Autodesk Fusion 360 part; units mm, degrees
(part 12 of 18)
sketch "Sketch4" plane through (0, 0, 3) normal (0, 0, 1) x (-1, 0, 0)
  arc A0 (-3.0787, 1.9914) -> (-3.5852, 0.7688) centre (0, 0) ccw
  line L0 (-3.5852, 0.7688) -> (-4.9003, 1.0509)
  line L1 (-4.9003, 1.0509) -> (-4.9011, 1.051)
  spline S0 degree 5 poles (-4.9011, 1.051) (-4.9011, 1.0511) (-4.9013, 1.0511) (-4.9016, 1.0512) (-4.9021, 1.0512) (-4.9028, 1.0514) (-4.9036, 1.0515) (-4.9045, 1.0517) (-4.9055, 1.0518) (-4.9066, 1.052) (-4.9078, 1.0522) (-4.9092, 1.0524) (-4.9106, 1.0526) (-4.9121, 1.0529) (-4.9137, 1.0531) (-4.9154, 1.0533) (-4.9172, 1.0536) (-4.9191, 1.0538) (-4.9211, 1.054) (-4.9232, 1.0543) (-4.9254, 1.0545) (-4.9277, 1.0548) (-4.9301, 1.055) (-4.9325, 1.0553) (-4.9351, 1.0555) (-4.9377, 1.0558) (-4.9404, 1.056) (-4.9432, 1.0562) (-4.9461, 1.0564) (-4.9491, 1.0567) (-4.9521, 1.0569) (-4.9553, 1.0571) (-4.9585, 1.0573) (-4.9618, 1.0575) (-4.9652, 1.0576) (-4.9687, 1.0578) (-4.9722, 1.058) (-4.9758, 1.0581) (-4.9795, 1.0582) (-4.9833, 1.0583) (-4.9872, 1.0584) (-4.9911, 1.0585) (-4.9951, 1.0586) (-4.9992, 1.0587) (-5.0033, 1.0587) (-5.0075, 1.0587) (-5.0118, 1.0587) (-5.0162, 1.0587) (-5.0206, 1.0587) (-5.0251, 1.0587) (-5.0297, 1.0586) (-5.0344, 1.0585) (-5.0391, 1.0584) (-5.0439, 1.0583) (-5.0487, 1.0581) (-5.0536, 1.058) (-5.0586, 1.0578) (-5.0637, 1.0576) (-5.0688, 1.0573) (-5.074, 1.0571) (-5.0792, 1.0568) (-5.0845, 1.0565) (-5.0899, 1.0561) (-5.0953, 1.0558) (-5.1008, 1.0554) (-5.1063, 1.055) (-5.112, 1.0545) (-5.1176, 1.0541) (-5.1234, 1.0536) (-5.1291, 1.0531) (-5.135, 1.0525) (-5.1409, 1.0519) (-5.1469, 1.0513) (-5.1529, 1.0507) (-5.159, 1.05) (-5.1651, 1.0493) (-5.1713, 1.0486) (-5.1775, 1.0479) (-5.1838, 1.0471) (-5.1902, 1.0463) (-5.1966, 1.0454) (-5.203, 1.0446) (-5.2095, 1.0436) (-5.2161, 1.0427) (-5.2227, 1.0417) (-5.2294, 1.0407) (-5.2361, 1.0397) (-5.2428, 1.0386) (-5.2496, 1.0375) (-5.2565, 1.0364) (-5.2634, 1.0352) (-5.2704, 1.034) (-5.2774, 1.0327) (-5.2844, 1.0314) (-5.2915, 1.0301) (-5.2987, 1.0288) (-5.3059, 1.0274) (-5.3131, 1.026) (-5.3204, 1.0245) (-5.3277, 1.023) (-5.3351, 1.0215) (-5.3425, 1.0199) (-5.3499, 1.0183) (-5.3574, 1.0167) (-5.365, 1.015) (-5.3726, 1.0133) (-5.3802, 1.0115) (-5.3879, 1.0097) (-5.3956, 1.0079) (-5.4033, 1.006) (-5.4111, 1.0041) (-5.4189, 1.0021) (-5.4268, 1.0001) (-5.4347, 0.9981) (-5.4427, 0.996) (-5.4506, 0.9939) (-5.4587, 0.9918) (-5.4667, 0.9896) (-5.4748, 0.9874) (-5.483, 0.9851) (-5.4911, 0.9828) (-5.4993, 0.9804) (-5.5076, 0.978) (-5.5159, 0.9756) (-5.5242, 0.9731) (-5.5325, 0.9706) (-5.5409, 0.968) (-5.5493, 0.9654) (-5.5577, 0.9628) (-5.5662, 0.9601) (-5.5747, 0.9574) (-5.5833, 0.9546) (-5.5919, 0.9518) (-5.6005, 0.9489) (-5.6091, 0.946) (-5.6178, 0.9431) (-5.6265, 0.9401) (-5.6352, 0.9371) (-5.644, 0.934) (-5.6528, 0.9309) (-5.6616, 0.9277) (-5.6704, 0.9245) (-5.6793, 0.9213) (-5.6882, 0.918) (-5.6971, 0.9146) (-5.7061, 0.9113) (-5.7151, 0.9078) (-5.7241, 0.9044) (-5.7331, 0.9008) (-5.7422, 0.8973) (-5.7513, 0.8937) (-5.7604, 0.89) (-5.7695, 0.8863) (-5.7787, 0.8826) (-5.7879, 0.8788) (-5.7971, 0.875) (-5.8063, 0.8711) (-5.8156, 0.8672) (-5.8249, 0.8632) (-5.8342, 0.8592) (-5.8435, 0.8551) (-5.8529, 0.851) (-5.8622, 0.8469) (-5.8716, 0.8427) (-5.881, 0.8384) (-5.8905, 0.8341) (-5.8999, 0.8298) (-5.9094, 0.8254) (-5.9189, 0.821) (-5.9284, 0.8165) (-5.938, 0.812) (-5.9475, 0.8074) (-5.9571, 0.8028) (-5.9667, 0.7981) (-5.9763, 0.7934) (-5.9859, 0.7887) (-5.9956, 0.7839) (-6.0052, 0.779) (-6.0149, 0.7741) (-6.0246, 0.7692) (-6.0343, 0.7642) (-6.044, 0.7591) (-6.0538, 0.754) (-6.0635, 0.7489) (-6.0733, 0.7437) (-6.0831, 0.7385) (-6.0929, 0.7332) (-6.1027, 0.7279) (-6.1126, 0.7225) (-6.1224, 0.7171) (-6.1323, 0.7116) (-6.1421, 0.7061) (-6.152, 0.7005) (-6.1619, 0.6949) (-6.1718, 0.6893) (-6.1818, 0.6836) (-6.1917, 0.6778) (-6.2016, 0.672) (-6.2116, 0.6661) (-6.2216, 0.6602) (-6.2316, 0.6543) (-6.2415, 0.6483) (-6.2515, 0.6423) (-6.2616, 0.6362) (-6.2716, 0.63) (-6.2816, 0.6238) (-6.2916, 0.6176) (-6.3017, 0.6113) (-6.3117, 0.605) (-6.3218, 0.5986) (-6.3319, 0.5921) (-6.342, 0.5857) (-6.3521, 0.5791) (-6.3621, 0.5726) (-6.3722, 0.5659) (-6.3824, 0.5593) (-6.3925, 0.5525) (-6.4026, 0.5458) (-6.4127, 0.5389) (-6.4229, 0.5321) (-6.433, 0.5252) (-6.4431, 0.5182) (-6.4533, 0.5112) (-6.4634, 0.5041) (-6.4736, 0.497) (-6.4838, 0.4898) (-6.4939, 0.4826) (-6.5041, 0.4754) (-6.5143, 0.4681) (-6.5244, 0.4607) (-6.5346, 0.4533) (-6.5448, 0.4459) (-6.555, 0.4384) (-6.5652, 0.4308) (-6.5754, 0.4232) (-6.5855, 0.4156) (-6.5957, 0.4079) (-6.6059, 0.4001) (-6.6161, 0.3923) (-6.6263, 0.3845) (-6.6365, 0.3766) (-6.6447, 0.3702) (-6.6508, 0.3655) (-6.6549, 0.3623) (-6.6569, 0.3607) knots 0 0 0 0 0 0 0.00416667 0.00833333 0.0125 0.01666667 0.02083333 0.025 0.02916667 0.03333333 0.0375 0.04166667 0.04583333 0.05 0.05416667 0.05833333 0.0625 0.06666667 0.07083333 0.075 0.07916667 0.08333333 0.0875 0.09166667 0.09583333 0.1 0.10416667 0.10833333 0.1125 0.11666667 0.12083333 0.125 0.12916667 0.13333333 0.1375 0.14166667 0.14583333 0.15 0.15416667 0.15833333 0.1625 0.16666667 0.17083333 0.175 0.17916667 0.18333333 0.1875 0.19166667 0.19583333 0.2 0.20416667 0.20833333 0.2125 0.21666667 0.22083333 0.225 0.22916667 0.23333333 0.2375 0.24166667 0.24583333 0.25 0.25416667 0.25833333 0.2625 0.26666667 0.27083333 0.275 0.27916667 0.28333333 0.2875 0.29166667 0.29583333 0.3 0.30416667 0.30833333 0.3125 0.31666667 0.32083333 0.325 0.32916667 0.33333333 0.3375 0.34166667 0.34583333 0.35 0.35416667 0.35833333 0.3625 0.36666667 0.37083333 0.375 0.37916667 0.38333333 0.3875 0.39166667 0.39583333 0.4 0.40416667 0.40833333 0.4125 0.41666667 0.42083333 0.425 0.42916667 0.43333333 0.4375 0.44166667 0.44583333 0.45 0.45416667 0.45833333 0.4625 0.46666667 0.47083333 0.475 0.47916667 0.48333333 0.4875 0.49166667 0.49583333 0.5 0.50416667 0.50833333 0.5125 0.51666667 0.52083333 0.525 0.52916667 0.53333333 0.5375 0.54166667 0.54583333 0.55 0.55416667 0.55833333 0.5625 0.56666667 0.57083333 0.575 0.57916667 0.58333333 0.5875 0.59166667 0.59583333 0.6 0.60416667 0.60833333 0.6125 0.61666667 0.62083333 0.625 0.62916667 0.63333333 0.6375 0.64166667 0.64583333 0.65 0.65416667 0.65833333 0.6625 0.66666667 0.67083333 0.675 0.67916667 0.68333333 0.6875 0.69166667 0.69583333 0.7 0.70416667 0.70833333 0.7125 0.71666667 0.72083333 0.725 0.72916667 0.73333333 0.7375 0.74166667 0.74583333 0.75 0.75416667 0.75833333 0.7625 0.76666667 0.77083333 0.775 0.77916667 0.78333333 0.7875 0.79166667 0.79583333 0.8 0.80416667 0.80833333 0.8125 0.81666667 0.82083333 0.825 0.82916667 0.83333333 0.8375 0.84166667 0.84583333 0.85 0.85416667 0.85833333 0.8625 0.86666667 0.87083333 0.875 0.87916667 0.88333333 0.8875 0.89166667 0.89583333 0.9 0.90416667 0.90833333 0.9125 0.91666667 0.92083333 0.925 0.92916667 0.93333333 0.9375 0.94166667 0.94583333 0.95 0.95416667 0.95833333 0.9625 0.96666667 0.97083333 0.975 0.97916667 0.98333333 0.9875 0.99166667 0.99583333 1 1 1 1 1 1
  arc A1 (-6.6569, 0.3607) -> (-6.6569, -0.3607) centre (0, 0) ccw
  spline S1 degree 5 poles (-6.6569, -0.3607) (-6.6549, -0.3623) (-6.6508, -0.3655) (-6.6447, -0.3702) (-6.6365, -0.3766) (-6.6263, -0.3845) (-6.6161, -0.3923) (-6.6059, -0.4001) (-6.5957, -0.4079) (-6.5855, -0.4156) (-6.5754, -0.4232) (-6.5652, -0.4308) (-6.555, -0.4384) (-6.5448, -0.4459) (-6.5346, -0.4533) (-6.5244, -0.4607) (-6.5143, -0.4681) (-6.5041, -0.4754) (-6.4939, -0.4826) (-6.4838, -0.4898) (-6.4736, -0.497) (-6.4634, -0.5041) (-6.4533, -0.5112) (-6.4431, -0.5182) (-6.433, -0.5252) (-6.4229, -0.5321) (-6.4127, -0.5389) (-6.4026, -0.5458) (-6.3925, -0.5525) (-6.3824, -0.5593) (-6.3722, -0.5659) (-6.3621, -0.5726) (-6.3521, -0.5791) (-6.342, -0.5857) (-6.3319, -0.5921) (-6.3218, -0.5986) (-6.3117, -0.605) (-6.3017, -0.6113) (-6.2916, -0.6176) (-6.2816, -0.6238) (-6.2716, -0.63) (-6.2616, -0.6362) (-6.2515, -0.6423) (-6.2415, -0.6483) (-6.2316, -0.6543) (-6.2216, -0.6602) (-6.2116, -0.6661) (-6.2016, -0.672) (-6.1917, -0.6778) (-6.1818, -0.6836) (-6.1718, -0.6893) (-6.1619, -0.6949) (-6.152, -0.7005) (-6.1421, -0.7061) (-6.1323, -0.7116) (-6.1224, -0.7171) (-6.1126, -0.7225) (-6.1027, -0.7279) (-6.0929, -0.7332) (-6.0831, -0.7385) (-6.0733, -0.7437) (-6.0635, -0.7489) (-6.0538, -0.754) (-6.044, -0.7591) (-6.0343, -0.7642) (-6.0246, -0.7692) (-6.0149, -0.7741) (-6.0052, -0.779) (-5.9956, -0.7839) (-5.9859, -0.7887) (-5.9763, -0.7934) (-5.9667, -0.7981) (-5.9571, -0.8028) (-5.9475, -0.8074) (-5.938, -0.812) (-5.9284, -0.8165) (-5.9189, -0.821) (-5.9094, -0.8254) (-5.8999, -0.8298) (-5.8905, -0.8341) (-5.881, -0.8384) (-5.8716, -0.8427) (-5.8622, -0.8469) (-5.8529, -0.851) (-5.8435, -0.8551) (-5.8342, -0.8592) (-5.8249, -0.8632) (-5.8156, -0.8672) (-5.8063, -0.8711) (-5.7971, -0.875) (-5.7879, -0.8788) (-5.7787, -0.8826) (-5.7695, -0.8863) (-5.7604, -0.89) (-5.7513, -0.8937) (-5.7422, -0.8973) (-5.7331, -0.9008) (-5.7241, -0.9044) (-5.7151, -0.9078) (-5.7061, -0.9113) (-5.6971, -0.9146) (-5.6882, -0.918) (-5.6793, -0.9213) (-5.6704, -0.9245) (-5.6616, -0.9277) (-5.6528, -0.9309) (-5.644, -0.934) (-5.6352, -0.9371) (-5.6265, -0.9401) (-5.6178, -0.9431) (-5.6091, -0.946) (-5.6005, -0.9489) (-5.5919, -0.9518) (-5.5833, -0.9546) (-5.5747, -0.9574) (-5.5662, -0.9601) (-5.5577, -0.9628) (-5.5493, -0.9654) (-5.5409, -0.968) (-5.5325, -0.9706) (-5.5242, -0.9731) (-5.5159, -0.9756) (-5.5076, -0.978) (-5.4993, -0.9804) (-5.4911, -0.9828) (-5.483, -0.9851) (-5.4748, -0.9874) (-5.4667, -0.9896) (-5.4587, -0.9918) (-5.4506, -0.9939) (-5.4427, -0.996) (-5.4347, -0.9981) (-5.4268, -1.0001) (-5.4189, -1.0021) (-5.4111, -1.0041) (-5.4033, -1.006) (-5.3956, -1.0079) (-5.3879, -1.0097) (-5.3802, -1.0115) (-5.3726, -1.0133) (-5.365, -1.015) (-5.3574, -1.0167) (-5.3499, -1.0183) (-5.3425, -1.0199) (-5.3351, -1.0215) (-5.3277, -1.023) (-5.3204, -1.0245) (-5.3131, -1.026) (-5.3059, -1.0274) (-5.2987, -1.0288) (-5.2915, -1.0301) (-5.2844, -1.0314) (-5.2774, -1.0327) (-5.2704, -1.034) (-5.2634, -1.0352) (-5.2565, -1.0364) (-5.2496, -1.0375) (-5.2428, -1.0386) (-5.2361, -1.0397) (-5.2294, -1.0407) (-5.2227, -1.0417) (-5.2161, -1.0427) (-5.2095, -1.0436) (-5.203, -1.0446) (-5.1966, -1.0454) (-5.1902, -1.0463) (-5.1838, -1.0471) (-5.1775, -1.0479) (-5.1713, -1.0486) (-5.1651, -1.0493) (-5.159, -1.05) (-5.1529, -1.0507) (-5.1469, -1.0513) (-5.1409, -1.0519) (-5.135, -1.0525) (-5.1291, -1.0531) (-5.1234, -1.0536) (-5.1176, -1.0541) (-5.112, -1.0545) (-5.1063, -1.055) (-5.1008, -1.0554) (-5.0953, -1.0558) (-5.0899, -1.0561) (-5.0845, -1.0565) (-5.0792, -1.0568) (-5.074, -1.0571) (-5.0688, -1.0573) (-5.0637, -1.0576) (-5.0586, -1.0578) (-5.0536, -1.058) (-5.0487, -1.0581) (-5.0439, -1.0583) (-5.0391, -1.0584) (-5.0344, -1.0585) (-5.0297, -1.0586) (-5.0251, -1.0587) (-5.0206, -1.0587) (-5.0162, -1.0587) (-5.0118, -1.0587) (-5.0075, -1.0587) (-5.0033, -1.0587) (-4.9992, -1.0587) (-4.9951, -1.0586) (-4.9911, -1.0585) (-4.9872, -1.0584) (-4.9833, -1.0583) (-4.9795, -1.0582) (-4.9758, -1.0581) (-4.9722, -1.058) (-4.9687, -1.0578) (-4.9652, -1.0576) (-4.9618, -1.0575) (-4.9585, -1.0573) (-4.9553, -1.0571) (-4.9521, -1.0569) (-4.9491, -1.0567) (-4.9461, -1.0564) (-4.9432, -1.0562) (-4.9404, -1.056) (-4.9377, -1.0558) (-4.9351, -1.0555) (-4.9325, -1.0553) (-4.9301, -1.055) (-4.9277, -1.0548) (-4.9254, -1.0545) (-4.9232, -1.0543) (-4.9211, -1.054) (-4.9191, -1.0538) (-4.9172, -1.0536) (-4.9154, -1.0533) (-4.9137, -1.0531) (-4.9121, -1.0529) (-4.9106, -1.0526) (-4.9092, -1.0524) (-4.9078, -1.0522) (-4.9066, -1.052) (-4.9055, -1.0518) (-4.9045, -1.0517) (-4.9036, -1.0515) (-4.9028, -1.0514) (-4.9021, -1.0512) (-4.9016, -1.0512) (-4.9013, -1.0511) (-4.9011, -1.0511) (-4.9011, -1.051) knots -1 -1 -1 -1 -1 -1 -0.99583333 -0.99166667 -0.9875 -0.98333333 -0.97916667 -0.975 -0.97083333 -0.96666667 -0.9625 -0.95833333 -0.95416667 -0.95 -0.94583333 -0.94166667 -0.9375 -0.93333333 -0.92916667 -0.925 -0.92083333 -0.91666667 -0.9125 -0.90833333 -0.90416667 -0.9 -0.89583333 -0.89166667 -0.8875 -0.88333333 -0.87916667 -0.875 -0.87083333 -0.86666667 -0.8625 -0.85833333 -0.85416667 -0.85 -0.84583333 -0.84166667 -0.8375 -0.83333333 -0.82916667 -0.825 -0.82083333 -0.81666667 -0.8125 -0.80833333 -0.80416667 -0.8 -0.79583333 -0.79166667 -0.7875 -0.78333333 -0.77916667 -0.775 -0.77083333 -0.76666667 -0.7625 -0.75833333 -0.75416667 -0.75 -0.74583333 -0.74166667 -0.7375 -0.73333333 -0.72916667 -0.725 -0.72083333 -0.71666667 -0.7125 -0.70833333 -0.70416667 -0.7 -0.69583333 -0.69166667 -0.6875 -0.68333333 -0.67916667 -0.675 -0.67083333 -0.66666667 -0.6625 -0.65833333 -0.65416667 -0.65 -0.64583333 -0.64166667 -0.6375 -0.63333333 -0.62916667 -0.625 -0.62083333 -0.61666667 -0.6125 -0.60833333 -0.60416667 -0.6 -0.59583333 -0.59166667 -0.5875 -0.58333333 -0.57916667 -0.575 -0.57083333 -0.56666667 -0.5625 -0.55833333 -0.55416667 -0.55 -0.54583333 -0.54166667 -0.5375 -0.53333333 -0.52916667 -0.525 -0.52083333 -0.51666667 -0.5125 -0.50833333 -0.50416667 -0.5 -0.49583333 -0.49166667 -0.4875 -0.48333333 -0.47916667 -0.475 -0.47083333 -0.46666667 -0.4625 -0.45833333 -0.45416667 -0.45 -0.44583333 -0.44166667 -0.4375 -0.43333333 -0.42916667 -0.425 -0.42083333 -0.41666667 -0.4125 -0.40833333 -0.40416667 -0.4 -0.39583333 -0.39166667 -0.3875 -0.38333333 -0.37916667 -0.375 -0.37083333 -0.36666667 -0.3625 -0.35833333 -0.35416667 -0.35 -0.34583333 -0.34166667 -0.3375 -0.33333333 -0.32916667 -0.325 -0.32083333 -0.31666667 -0.3125 -0.30833333 -0.30416667 -0.3 -0.29583333 -0.29166667 -0.2875 -0.28333333 -0.27916667 -0.275 -0.27083333 -0.26666667 -0.2625 -0.25833333 -0.25416667 -0.25 -0.24583333 -0.24166667 -0.2375 -0.23333333 -0.22916667 -0.225 -0.22083333 -0.21666667 -0.2125 -0.20833333 -0.20416667 -0.2 -0.19583333 -0.19166667 -0.1875 -0.18333333 -0.17916667 -0.175 -0.17083333 -0.16666667 -0.1625 -0.15833333 -0.15416667 -0.15 -0.14583333 -0.14166667 -0.1375 -0.13333333 -0.12916667 -0.125 -0.12083333 -0.11666667 -0.1125 -0.10833333 -0.10416667 -0.1 -0.09583333 -0.09166667 -0.0875 -0.08333333 -0.07916667 -0.075 -0.07083333 -0.06666667 -0.0625 -0.05833333 -0.05416667 -0.05 -0.04583333 -0.04166667 -0.0375 -0.03333333 -0.02916667 -0.025 -0.02083333 -0.01666667 -0.0125 -0.00833333 -0.00416667 0 0 0 0 0 0
  line L2 (-4.9011, -1.051) -> (-4.9003, -1.0509)
  line L3 (-4.9003, -1.0509) -> (-3.5852, -0.7688)
  arc A2 (-3.5852, -0.7688) -> (-3.0787, -1.9914) centre (0, 0) ccw
  line L4 (-3.0787, -1.9914) -> (-4.2081, -2.7219)
  line L5 (-4.2081, -2.7219) -> (-4.2088, -2.7224)
  spline S2 degree 5 poles (-4.2088, -2.7224) (-4.2088, -2.7224) (-4.209, -2.7225) (-4.2093, -2.7227) (-4.2096, -2.723) (-4.2102, -2.7234) (-4.2109, -2.7238) (-4.2116, -2.7244) (-4.2125, -2.725) (-4.2134, -2.7256) (-4.2144, -2.7263) (-4.2155, -2.7271) (-4.2166, -2.728) (-4.2179, -2.7289) (-4.2192, -2.7299) (-4.2205, -2.7309) (-4.222, -2.732) (-4.2235, -2.7332) (-4.2251, -2.7345) (-4.2267, -2.7358) (-4.2285, -2.7371) (-4.2302, -2.7386) (-4.2321, -2.7401) (-4.234, -2.7416) (-4.236, -2.7433) (-4.238, -2.7449) (-4.2401, -2.7467) (-4.2422, -2.7485) (-4.2444, -2.7504) (-4.2467, -2.7524) (-4.249, -2.7544) (-4.2514, -2.7564) (-4.2538, -2.7586) (-4.2563, -2.7608) (-4.2588, -2.7631) (-4.2613, -2.7654) (-4.264, -2.7678) (-4.2666, -2.7702) (-4.2693, -2.7728) (-4.2721, -2.7754) (-4.2749, -2.778) (-4.2777, -2.7807) (-4.2806, -2.7835) (-4.2835, -2.7863) (-4.2865, -2.7893) (-4.2895, -2.7922) (-4.2925, -2.7953) (-4.2956, -2.7984) (-4.2987, -2.8015) (-4.3019, -2.8047) (-4.3051, -2.808) (-4.3083, -2.8114) (-4.3116, -2.8148) (-4.3149, -2.8182) (-4.3182, -2.8218) (-4.3216, -2.8254) (-4.3249, -2.829) (-4.3284, -2.8328) (-4.3318, -2.8365) (-4.3353, -2.8404) (-4.3388, -2.8443) (-4.3423, -2.8483) (-4.3459, -2.8523) (-4.3495, -2.8564) (-4.3531, -2.8605) (-4.3567, -2.8648) (-4.3604, -2.869) (-4.364, -2.8734) (-4.3678, -2.8778) (-4.3715, -2.8822) (-4.3752, -2.8867) (-4.379, -2.8913) (-4.3828, -2.896) (-4.3866, -2.9007) (-4.3904, -2.9054) (-4.3943, -2.9103) (-4.3981, -2.9152) (-4.402, -2.9201) (-4.4059, -2.9251) (-4.4098, -2.9302) (-4.4138, -2.9353) (-4.4177, -2.9405) (-4.4217, -2.9457) (-4.4256, -2.951) (-4.4296, -2.9564) (-4.4336, -2.9618) (-4.4376, -2.9673) (-4.4416, -2.9728) (-4.4457, -2.9784) (-4.4497, -2.9841) (-4.4538, -2.9898) (-4.4578, -2.9956) (-4.4619, -3.0014) (-4.466, -3.0073) (-4.4701, -3.0133) (-4.4742, -3.0193) (-4.4783, -3.0253) (-4.4824, -3.0314) (-4.4865, -3.0376) (-4.4906, -3.0439) (-4.4948, -3.0502) (-4.4989, -3.0565) (-4.503, -3.0629) (-4.5072, -3.0694) (-4.5113, -3.0759) (-4.5155, -3.0825) (-4.5196, -3.0891) (-4.5238, -3.0958) (-4.5279, -3.1026) (-4.5321, -3.1094) (-4.5362, -3.1162) (-4.5404, -3.1231) (-4.5445, -3.1301) (-4.5487, -3.1371) (-4.5529, -3.1442) (-4.557, -3.1514) (-4.5612, -3.1586) (-4.5653, -3.1658) (-4.5695, -3.1731) (-4.5736, -3.1805) (-4.5777, -3.1879) (-4.5819, -3.1953) (-4.586, -3.2029) (-4.5902, -3.2104) (-4.5943, -3.2181) (-4.5984, -3.2258) (-4.6025, -3.2335) (-4.6066, -3.2413) (-4.6107, -3.2491) (-4.6148, -3.257) (-4.6189, -3.265) (-4.623, -3.273) (-4.6271, -3.281) (-4.6311, -3.2891) (-4.6352, -3.2973) (-4.6392, -3.3055) (-4.6433, -3.3138) (-4.6473, -3.3221) (-4.6513, -3.3304) (-4.6553, -3.3389) (-4.6593, -3.3473) (-4.6633, -3.3559) (-4.6673, -3.3644) (-4.6713, -3.3731) (-4.6752, -3.3817) (-4.6792, -3.3905) (-4.6831, -3.3992) (-4.687, -3.4081) (-4.6909, -3.4169) (-4.6948, -3.4259) (-4.6987, -3.4348) (-4.7026, -3.4439) (-4.7064, -3.4529) (-4.7102, -3.4621) (-4.7141, -3.4712) (-4.7179, -3.4805) (-4.7217, -3.4897) (-4.7254, -3.4991) (-4.7292, -3.5084) (-4.7329, -3.5178) (-4.7367, -3.5273) (-4.7404, -3.5368) (-4.7441, -3.5464) (-4.7477, -3.556) (-4.7514, -3.5657) (-4.755, -3.5754) (-4.7586, -3.5851) (-4.7622, -3.5949) (-4.7658, -3.6048) (-4.7694, -3.6147) (-4.7729, -3.6246) (-4.7765, -3.6346) (-4.78, -3.6446) (-4.7834, -3.6547) (-4.7869, -3.6648) (-4.7904, -3.675) (-4.7938, -3.6852) (-4.7972, -3.6955) (-4.8006, -3.7058) (-4.8039, -3.7161) (-4.8073, -3.7265) (-4.8106, -3.737) (-4.8139, -3.7475) (-4.8171, -3.758) (-4.8204, -3.7686) (-4.8236, -3.7792) (-4.8268, -3.7899) (-4.83, -3.8006) (-4.8331, -3.8113) (-4.8363, -3.8221) (-4.8394, -3.833) (-4.8424, -3.8439) (-4.8455, -3.8548) (-4.8485, -3.8658) (-4.8515, -3.8768) (-4.8545, -3.8878) (-4.8575, -3.8989) (-4.8604, -3.9101) (-4.8633, -3.9212) (-4.8662, -3.9325) (-4.869, -3.9437) (-4.8719, -3.955) (-4.8747, -3.9664) (-4.8774, -3.9778) (-4.8802, -3.9892) (-4.8829, -4.0007) (-4.8856, -4.0122) (-4.8882, -4.0237) (-4.8909, -4.0353) (-4.8935, -4.0469) (-4.896, -4.0586) (-4.8986, -4.0703) (-4.9011, -4.0821) (-4.9036, -4.0939) (-4.906, -4.1057) (-4.9085, -4.1176) (-4.9109, -4.1295) (-4.9132, -4.1414) (-4.9156, -4.1534) (-4.9179, -4.1654) (-4.9201, -4.1775) (-4.9224, -4.1896) (-4.9246, -4.2017) (-4.9268, -4.2139) (-4.9289, -4.2261) (-4.9311, -4.2383) (-4.9332, -4.2506) (-4.9352, -4.2629) (-4.9372, -4.2753) (-4.9392, -4.2877) (-4.9412, -4.3001) (-4.9431, -4.3126) (-4.945, -4.3251) (-4.9469, -4.3377) (-4.9487, -4.3502) (-4.9505, -4.3628) (-4.9523, -4.3755) (-4.954, -4.3882) (-4.9557, -4.4009) (-4.9574, -4.4136) (-4.959, -4.4264) (-4.9603, -4.4367) (-4.9612, -4.4444) (-4.9619, -4.4495) (-4.9622, -4.4521) knots 0 0 0 0 0 0 0.00416667 0.00833333 0.0125 0.01666667 0.02083333 0.025 0.02916667 0.03333333 0.0375 0.04166667 0.04583333 0.05 0.05416667 0.05833333 0.0625 0.06666667 0.07083333 0.075 0.07916667 0.08333333 0.0875 0.09166667 0.09583333 0.1 0.10416667 0.10833333 0.1125 0.11666667 0.12083333 0.125 0.12916667 0.13333333 0.1375 0.14166667 0.14583333 0.15 0.15416667 0.15833333 0.1625 0.16666667 0.17083333 0.175 0.17916667 0.18333333 0.1875 0.19166667 0.19583333 0.2 0.20416667 0.20833333 0.2125 0.21666667 0.22083333 0.225 0.22916667 0.23333333 0.2375 0.24166667 0.24583333 0.25 0.25416667 0.25833333 0.2625 0.26666667 0.27083333 0.275 0.27916667 0.28333333 0.2875 0.29166667 0.29583333 0.3 0.30416667 0.30833333 0.3125 0.31666667 0.32083333 0.325 0.32916667 0.33333333 0.3375 0.34166667 0.34583333 0.35 0.35416667 0.35833333 0.3625 0.36666667 0.37083333 0.375 0.37916667 0.38333333 0.3875 0.39166667 0.39583333 0.4 0.40416667 0.40833333 0.4125 0.41666667 0.42083333 0.425 0.42916667 0.43333333 0.4375 0.44166667 0.44583333 0.45 0.45416667 0.45833333 0.4625 0.46666667 0.47083333 0.475 0.47916667 0.48333333 0.4875 0.49166667 0.49583333 0.5 0.50416667 0.50833333 0.5125 0.51666667 0.52083333 0.525 0.52916667 0.53333333 0.5375 0.54166667 0.54583333 0.55 0.55416667 0.55833333 0.5625 0.56666667 0.57083333 0.575 0.57916667 0.58333333 0.5875 0.59166667 0.59583333 0.6 0.60416667 0.60833333 0.6125 0.61666667 0.62083333 0.625 0.62916667 0.63333333 0.6375 0.64166667 0.64583333 0.65 0.65416667 0.65833333 0.6625 0.66666667 0.67083333 0.675 0.67916667 0.68333333 0.6875 0.69166667 0.69583333 0.7 0.70416667 0.70833333 0.7125 0.71666667 0.72083333 0.725 0.72916667 0.73333333 0.7375 0.74166667 0.74583333 0.75 0.75416667 0.75833333 0.7625 0.76666667 0.77083333 0.775 0.77916667 0.78333333 0.7875 0.79166667 0.79583333 0.8 0.80416667 0.80833333 0.8125 0.81666667 0.82083333 0.825 0.82916667 0.83333333 0.8375 0.84166667 0.84583333 0.85 0.85416667 0.85833333 0.8625 0.86666667 0.87083333 0.875 0.87916667 0.88333333 0.8875 0.89166667 0.89583333 0.9 0.90416667 0.90833333 0.9125 0.91666667 0.92083333 0.925 0.92916667 0.93333333 0.9375 0.94166667 0.94583333 0.95 0.95416667 0.95833333 0.9625 0.96666667 0.97083333 0.975 0.97916667 0.98333333 0.9875 0.99166667 0.99583333 1 1 1 1 1 1
  arc A3 (-4.9622, -4.4521) -> (-4.4521, -4.9622) centre (0, 0) ccw
  spline S3 degree 5 poles (-4.4521, -4.9622) (-4.4495, -4.9619) (-4.4444, -4.9612) (-4.4367, -4.9603) (-4.4264, -4.959) (-4.4136, -4.9574) (-4.4009, -4.9557) (-4.3882, -4.954) (-4.3755, -4.9523) (-4.3628, -4.9505) (-4.3502, -4.9487) (-4.3377, -4.9469) (-4.3251, -4.945) (-4.3126, -4.9431) (-4.3001, -4.9412) (-4.2877, -4.9392) (-4.2753, -4.9372) (-4.2629, -4.9352) (-4.2506, -4.9332) (-4.2383, -4.9311) (-4.2261, -4.9289) (-4.2139, -4.9268) (-4.2017, -4.9246) (-4.1896, -4.9224) (-4.1775, -4.9201) (-4.1654, -4.9179) (-4.1534, -4.9156) (-4.1414, -4.9132) (-4.1295, -4.9109) (-4.1176, -4.9085) (-4.1057, -4.906) (-4.0939, -4.9036) (-4.0821, -4.9011) (-4.0703, -4.8986) (-4.0586, -4.896) (-4.0469, -4.8935) (-4.0353, -4.8909) (-4.0237, -4.8882) (-4.0122, -4.8856) (-4.0007, -4.8829) (-3.9892, -4.8802) (-3.9778, -4.8774) (-3.9664, -4.8747) (-3.955, -4.8719) (-3.9437, -4.869) (-3.9325, -4.8662) (-3.9212, -4.8633) (-3.9101, -4.8604) (-3.8989, -4.8575) (-3.8878, -4.8545) (-3.8768, -4.8515) (-3.8658, -4.8485) (-3.8548, -4.8455) (-3.8439, -4.8424) (-3.833, -4.8394) (-3.8221, -4.8363) (-3.8113, -4.8331) (-3.8006, -4.83) (-3.7899, -4.8268) (-3.7792, -4.8236) (-3.7686, -4.8204) (-3.758, -4.8171) (-3.7475, -4.8139) (-3.737, -4.8106) (-3.7265, -4.8073) (-3.7161, -4.8039) (-3.7058, -4.8006) (-3.6955, -4.7972) (-3.6852, -4.7938) (-3.675, -4.7904) (-3.6648, -4.7869) (-3.6547, -4.7834) (-3.6446, -4.78) (-3.6346, -4.7765) (-3.6246, -4.7729) (-3.6147, -4.7694) (-3.6048, -4.7658) (-3.5949, -4.7622) (-3.5851, -4.7586) (-3.5754, -4.755) (-3.5657, -4.7514) (-3.556, -4.7477) (-3.5464, -4.7441) (-3.5368, -4.7404) (-3.5273, -4.7367) (-3.5178, -4.7329) (-3.5084, -4.7292) (-3.4991, -4.7254) (-3.4897, -4.7217) (-3.4805, -4.7179) (-3.4712, -4.7141) (-3.4621, -4.7102) (-3.4529, -4.7064) (-3.4439, -4.7026) (-3.4348, -4.6987) (-3.4259, -4.6948) (-3.4169, -4.6909) (-3.4081, -4.687) (-3.3992, -4.6831) (-3.3905, -4.6792) (-3.3817, -4.6752) (-3.3731, -4.6713) (-3.3644, -4.6673) (-3.3559, -4.6633) (-3.3473, -4.6593) (-3.3389, -4.6553) (-3.3304, -4.6513) (-3.3221, -4.6473) (-3.3138, -4.6433) (-3.3055, -4.6392) (-3.2973, -4.6352) (-3.2891, -4.6311) (-3.281, -4.6271) (-3.273, -4.623) (-3.265, -4.6189) (-3.257, -4.6148) (-3.2491, -4.6107) (-3.2413, -4.6066) (-3.2335, -4.6025) (-3.2258, -4.5984) (-3.2181, -4.5943) (-3.2104, -4.5902) (-3.2029, -4.586) (-3.1953, -4.5819) (-3.1879, -4.5777) (-3.1805, -4.5736) (-3.1731, -4.5695) (-3.1658, -4.5653) (-3.1586, -4.5612) (-3.1514, -4.557) (-3.1442, -4.5529) (-3.1371, -4.5487) (-3.1301, -4.5445) (-3.1231, -4.5404) (-3.1162, -4.5362) (-3.1094, -4.5321) (-3.1026, -4.5279) (-3.0958, -4.5238) (-3.0891, -4.5196) (-3.0825, -4.5155) (-3.0759, -4.5113) (-3.0694, -4.5072) (-3.0629, -4.503) (-3.0565, -4.4989) (-3.0502, -4.4948) (-3.0439, -4.4906) (-3.0376, -4.4865) (-3.0314, -4.4824) (-3.0253, -4.4783) (-3.0193, -4.4742) (-3.0133, -4.4701) (-3.0073, -4.466) (-3.0014, -4.4619) (-2.9956, -4.4578) (-2.9898, -4.4538) (-2.9841, -4.4497) (-2.9784, -4.4457) (-2.9728, -4.4416) (-2.9673, -4.4376) (-2.9618, -4.4336) (-2.9564, -4.4296) (-2.951, -4.4256) (-2.9457, -4.4217) (-2.9405, -4.4177) (-2.9353, -4.4138) (-2.9302, -4.4098) (-2.9251, -4.4059) (-2.9201, -4.402) (-2.9152, -4.3981) (-2.9103, -4.3943) (-2.9054, -4.3904) (-2.9007, -4.3866) (-2.896, -4.3828) (-2.8913, -4.379) (-2.8867, -4.3752) (-2.8822, -4.3715) (-2.8778, -4.3678) (-2.8734, -4.364) (-2.869, -4.3604) (-2.8648, -4.3567) (-2.8605, -4.3531) (-2.8564, -4.3495) (-2.8523, -4.3459) (-2.8483, -4.3423) (-2.8443, -4.3388) (-2.8404, -4.3353) (-2.8365, -4.3318) (-2.8328, -4.3284) (-2.829, -4.3249) (-2.8254, -4.3216) (-2.8218, -4.3182) (-2.8182, -4.3149) (-2.8148, -4.3116) (-2.8114, -4.3083) (-2.808, -4.3051) (-2.8047, -4.3019) (-2.8015, -4.2987) (-2.7984, -4.2956) (-2.7953, -4.2925) (-2.7922, -4.2895) (-2.7893, -4.2865) (-2.7863, -4.2835) (-2.7835, -4.2806) (-2.7807, -4.2777) (-2.778, -4.2749) (-2.7754, -4.2721) (-2.7728, -4.2693) (-2.7702, -4.2666) (-2.7678, -4.264) (-2.7654, -4.2613) (-2.7631, -4.2588) (-2.7608, -4.2563) (-2.7586, -4.2538) (-2.7564, -4.2514) (-2.7544, -4.249) (-2.7524, -4.2467) (-2.7504, -4.2444) (-2.7485, -4.2422) (-2.7467, -4.2401) (-2.7449, -4.238) (-2.7433, -4.236) (-2.7416, -4.234) (-2.7401, -4.2321) (-2.7386, -4.2302) (-2.7371, -4.2285) (-2.7358, -4.2267) (-2.7345, -4.2251) (-2.7332, -4.2235) (-2.732, -4.222) (-2.7309, -4.2205) (-2.7299, -4.2192) (-2.7289, -4.2179) (-2.728, -4.2166) (-2.7271, -4.2155) (-2.7263, -4.2144) (-2.7256, -4.2134) (-2.725, -4.2125) (-2.7244, -4.2116) (-2.7238, -4.2109) (-2.7234, -4.2102) (-2.723, -4.2096) (-2.7227, -4.2093) (-2.7225, -4.209) (-2.7224, -4.2088) (-2.7224, -4.2088) knots -1 -1 -1 -1 -1 -1 -0.99583333 -0.99166667 -0.9875 -0.98333333 -0.97916667 -0.975 -0.97083333 -0.96666667 -0.9625 -0.95833333 -0.95416667 -0.95 -0.94583333 -0.94166667 -0.9375 -0.93333333 -0.92916667 -0.925 -0.92083333 -0.91666667 -0.9125 -0.90833333 -0.90416667 -0.9 -0.89583333 -0.89166667 -0.8875 -0.88333333 -0.87916667 -0.875 -0.87083333 -0.86666667 -0.8625 -0.85833333 -0.85416667 -0.85 -0.84583333 -0.84166667 -0.8375 -0.83333333 -0.82916667 -0.825 -0.82083333 -0.81666667 -0.8125 -0.80833333 -0.80416667 -0.8 -0.79583333 -0.79166667 -0.7875 -0.78333333 -0.77916667 -0.775 -0.77083333 -0.76666667 -0.7625 -0.75833333 -0.75416667 -0.75 -0.74583333 -0.74166667 -0.7375 -0.73333333 -0.72916667 -0.725 -0.72083333 -0.71666667 -0.7125 -0.70833333 -0.70416667 -0.7 -0.69583333 -0.69166667 -0.6875 -0.68333333 -0.67916667 -0.675 -0.67083333 -0.66666667 -0.6625 -0.65833333 -0.65416667 -0.65 -0.64583333 -0.64166667 -0.6375 -0.63333333 -0.62916667 -0.625 -0.62083333 -0.61666667 -0.6125 -0.60833333 -0.60416667 -0.6 -0.59583333 -0.59166667 -0.5875 -0.58333333 -0.57916667 -0.575 -0.57083333 -0.56666667 -0.5625 -0.55833333 -0.55416667 -0.55 -0.54583333 -0.54166667 -0.5375 -0.53333333 -0.52916667 -0.525 -0.52083333 -0.51666667 -0.5125 -0.50833333 -0.50416667 -0.5 -0.49583333 -0.49166667 -0.4875 -0.48333333 -0.47916667 -0.475 -0.47083333 -0.46666667 -0.4625 -0.45833333 -0.45416667 -0.45 -0.44583333 -0.44166667 -0.4375 -0.43333333 -0.42916667 -0.425 -0.42083333 -0.41666667 -0.4125 -0.40833333 -0.40416667 -0.4 -0.39583333 -0.39166667 -0.3875 -0.38333333 -0.37916667 -0.375 -0.37083333 -0.36666667 -0.3625 -0.35833333 -0.35416667 -0.35 -0.34583333 -0.34166667 -0.3375 -0.33333333 -0.32916667 -0.325 -0.32083333 -0.31666667 -0.3125 -0.30833333 -0.30416667 -0.3 -0.29583333 -0.29166667 -0.2875 -0.28333333 -0.27916667 -0.275 -0.27083333 -0.26666667 -0.2625 -0.25833333 -0.25416667 -0.25 -0.24583333 -0.24166667 -0.2375 -0.23333333 -0.22916667 -0.225 -0.22083333 -0.21666667 -0.2125 -0.20833333 -0.20416667 -0.2 -0.19583333 -0.19166667 -0.1875 -0.18333333 -0.17916667 -0.175 -0.17083333 -0.16666667 -0.1625 -0.15833333 -0.15416667 -0.15 -0.14583333 -0.14166667 -0.1375 -0.13333333 -0.12916667 -0.125 -0.12083333 -0.11666667 -0.1125 -0.10833333 -0.10416667 -0.1 -0.09583333 -0.09166667 -0.0875 -0.08333333 -0.07916667 -0.075 -0.07083333 -0.06666667 -0.0625 -0.05833333 -0.05416667 -0.05 -0.04583333 -0.04166667 -0.0375 -0.03333333 -0.02916667 -0.025 -0.02083333 -0.01666667 -0.0125 -0.00833333 -0.00416667 0 0 0 0 0 0
  line L6 (-2.7224, -4.2088) -> (-2.7219, -4.2081)
  line L7 (-2.7219, -4.2081) -> (-1.9914, -3.0787)
  arc A4 (-1.9914, -3.0787) -> (-0.7688, -3.5852) centre (0, 0) ccw
  line L8 (-0.7688, -3.5852) -> (-1.0509, -4.9003)
  line L9 (-1.0509, -4.9003) -> (-1.051, -4.9011)
  spline S4 degree 5 poles (-1.051, -4.9011) (-1.0511, -4.9011) (-1.0511, -4.9013) (-1.0512, -4.9016) (-1.0512, -4.9021) (-1.0514, -4.9028) (-1.0515, -4.9036) (-1.0517, -4.9045) (-1.0518, -4.9055) (-1.052, -4.9066) (-1.0522, -4.9078) (-1.0524, -4.9092) (-1.0526, -4.9106) (-1.0529, -4.9121) (-1.0531, -4.9137) (-1.0533, -4.9154) (-1.0536, -4.9172) (-1.0538, -4.9191) (-1.054, -4.9211) (-1.0543, -4.9232) (-1.0545, -4.9254) (-1.0548, -4.9277) (-1.055, -4.9301) (-1.0553, -4.9325) (-1.0555, -4.9351) (-1.0558, -4.9377) (-1.056, -4.9404) (-1.0562, -4.9432) (-1.0564, -4.9461) (-1.0567, -4.9491) (-1.0569, -4.9521) (-1.0571, -4.9553) (-1.0573, -4.9585) (-1.0575, -4.9618) (-1.0576, -4.9652) (-1.0578, -4.9687) (-1.058, -4.9722) (-1.0581, -4.9758) (-1.0582, -4.9795) (-1.0583, -4.9833) (-1.0584, -4.9872) (-1.0585, -4.9911) (-1.0586, -4.9951) (-1.0587, -4.9992) (-1.0587, -5.0033) (-1.0587, -5.0075) (-1.0587, -5.0118) (-1.0587, -5.0162) (-1.0587, -5.0206) (-1.0587, -5.0251) (-1.0586, -5.0297) (-1.0585, -5.0344) (-1.0584, -5.0391) (-1.0583, -5.0439) (-1.0581, -5.0487) (-1.058, -5.0536) (-1.0578, -5.0586) (-1.0576, -5.0637) (-1.0573, -5.0688) (-1.0571, -5.074) (-1.0568, -5.0792) (-1.0565, -5.0845) (-1.0561, -5.0899) (-1.0558, -5.0953) (-1.0554, -5.1008) (-1.055, -5.1063) (-1.0545, -5.112) (-1.0541, -5.1176) (-1.0536, -5.1234) (-1.0531, -5.1291) (-1.0525, -5.135) (-1.0519, -5.1409) (-1.0513, -5.1469) (-1.0507, -5.1529) (-1.05, -5.159) (-1.0493, -5.1651) (-1.0486, -5.1713) (-1.0479, -5.1775) (-1.0471, -5.1838) (-1.0463, -5.1902) (-1.0454, -5.1966) (-1.0446, -5.203) (-1.0436, -5.2095) (-1.0427, -5.2161) (-1.0417, -5.2227) (-1.0407, -5.2294) (-1.0397, -5.2361) (-1.0386, -5.2428) (-1.0375, -5.2496) (-1.0364, -5.2565) (-1.0352, -5.2634) (-1.034, -5.2704) (-1.0327, -5.2774) (-1.0314, -5.2844) (-1.0301, -5.2915) (-1.0288, -5.2987) (-1.0274, -5.3059) (-1.026, -5.3131) (-1.0245, -5.3204) (-1.023, -5.3277) (-1.0215, -5.3351) (-1.0199, -5.3425) (-1.0183, -5.3499) (-1.0167, -5.3574) (-1.015, -5.365) (-1.0133, -5.3726) (-1.0115, -5.3802) (-1.0097, -5.3879) (-1.0079, -5.3956) (-1.006, -5.4033) (-1.0041, -5.4111) (-1.0021, -5.4189) (-1.0001, -5.4268) (-0.9981, -5.4347) (-0.996, -5.4427) (-0.9939, -5.4506) (-0.9918, -5.4587) (-0.9896, -5.4667) (-0.9874, -5.4748) (-0.9851, -5.483) (-0.9828, -5.4911) (-0.9804, -5.4993) (-0.978, -5.5076) (-0.9756, -5.5159) (-0.9731, -5.5242) (-0.9706, -5.5325) (-0.968, -5.5409) (-0.9654, -5.5493) (-0.9628, -5.5577) (-0.9601, -5.5662) (-0.9574, -5.5747) (-0.9546, -5.5833) (-0.9518, -5.5919) (-0.9489, -5.6005) (-0.946, -5.6091) (-0.9431, -5.6178) (-0.9401, -5.6265) (-0.9371, -5.6352) (-0.934, -5.644) (-0.9309, -5.6528) (-0.9277, -5.6616) (-0.9245, -5.6704) (-0.9213, -5.6793) (-0.918, -5.6882) (-0.9146, -5.6971) (-0.9113, -5.7061) (-0.9078, -5.7151) (-0.9044, -5.7241) (-0.9008, -5.7331) (-0.8973, -5.7422) (-0.8937, -5.7513) (-0.89, -5.7604) (-0.8863, -5.7695) (-0.8826, -5.7787) (-0.8788, -5.7879) (-0.875, -5.7971) (-0.8711, -5.8063) (-0.8672, -5.8156) (-0.8632, -5.8249) (-0.8592, -5.8342) (-0.8551, -5.8435) (-0.851, -5.8529) (-0.8469, -5.8622) (-0.8427, -5.8716) (-0.8384, -5.881) (-0.8341, -5.8905) (-0.8298, -5.8999) (-0.8254, -5.9094) (-0.821, -5.9189) (-0.8165, -5.9284) (-0.812, -5.938) (-0.8074, -5.9475) (-0.8028, -5.9571) (-0.7981, -5.9667) (-0.7934, -5.9763) (-0.7887, -5.9859) (-0.7839, -5.9956) (-0.779, -6.0052) (-0.7741, -6.0149) (-0.7692, -6.0246) (-0.7642, -6.0343) (-0.7591, -6.044) (-0.754, -6.0538) (-0.7489, -6.0635) (-0.7437, -6.0733) (-0.7385, -6.0831) (-0.7332, -6.0929) (-0.7279, -6.1027) (-0.7225, -6.1126) (-0.7171, -6.1224) (-0.7116, -6.1323) (-0.7061, -6.1421) (-0.7005, -6.152) (-0.6949, -6.1619) (-0.6893, -6.1718) (-0.6836, -6.1818) (-0.6778, -6.1917) (-0.672, -6.2016) (-0.6661, -6.2116) (-0.6602, -6.2216) (-0.6543, -6.2316) (-0.6483, -6.2415) (-0.6423, -6.2515) (-0.6362, -6.2616) (-0.63, -6.2716) (-0.6238, -6.2816) (-0.6176, -6.2916) (-0.6113, -6.3017) (-0.605, -6.3117) (-0.5986, -6.3218) (-0.5921, -6.3319) (-0.5857, -6.342) (-0.5791, -6.3521) (-0.5726, -6.3621) (-0.5659, -6.3722) (-0.5593, -6.3824) (-0.5525, -6.3925) (-0.5458, -6.4026) (-0.5389, -6.4127) (-0.5321, -6.4229) (-0.5252, -6.433) (-0.5182, -6.4431) (-0.5112, -6.4533) (-0.5041, -6.4634) (-0.497, -6.4736) (-0.4898, -6.4838) (-0.4826, -6.4939) (-0.4754, -6.5041) (-0.4681, -6.5143) (-0.4607, -6.5244) (-0.4533, -6.5346) (-0.4459, -6.5448) (-0.4384, -6.555) (-0.4308, -6.5652) (-0.4232, -6.5754) (-0.4156, -6.5855) (-0.4079, -6.5957) (-0.4001, -6.6059) (-0.3923, -6.6161) (-0.3845, -6.6263) (-0.3766, -6.6365) (-0.3702, -6.6447) (-0.3655, -6.6508) (-0.3623, -6.6549) (-0.3607, -6.6569) knots 0 0 0 0 0 0 0.00416667 0.00833333 0.0125 0.01666667 0.02083333 0.025 0.02916667 0.03333333 0.0375 0.04166667 0.04583333 0.05 0.05416667 0.05833333 0.0625 0.06666667 0.07083333 0.075 0.07916667 0.08333333 0.0875 0.09166667 0.09583333 0.1 0.10416667 0.10833333 0.1125 0.11666667 0.12083333 0.125 0.12916667 0.13333333 0.1375 0.14166667 0.14583333 0.15 0.15416667 0.15833333 0.1625 0.16666667 0.17083333 0.175 0.17916667 0.18333333 0.1875 0.19166667 0.19583333 0.2 0.20416667 0.20833333 0.2125 0.21666667 0.22083333 0.225 0.22916667 0.23333333 0.2375 0.24166667 0.24583333 0.25 0.25416667 0.25833333 0.2625 0.26666667 0.27083333 0.275 0.27916667 0.28333333 0.2875 0.29166667 0.29583333 0.3 0.30416667 0.30833333 0.3125 0.31666667 0.32083333 0.325 0.32916667 0.33333333 0.3375 0.34166667 0.34583333 0.35 0.35416667 0.35833333 0.3625 0.36666667 0.37083333 0.375 0.37916667 0.38333333 0.3875 0.39166667 0.39583333 0.4 0.40416667 0.40833333 0.4125 0.41666667 0.42083333 0.425 0.42916667 0.43333333 0.4375 0.44166667 0.44583333 0.45 0.45416667 0.45833333 0.4625 0.46666667 0.47083333 0.475 0.47916667 0.48333333 0.4875 0.49166667 0.49583333 0.5 0.50416667 0.50833333 0.5125 0.51666667 0.52083333 0.525 0.52916667 0.53333333 0.5375 0.54166667 0.54583333 0.55 0.55416667 0.55833333 0.5625 0.56666667 0.57083333 0.575 0.57916667 0.58333333 0.5875 0.59166667 0.59583333 0.6 0.60416667 0.60833333 0.6125 0.61666667 0.62083333 0.625 0.62916667 0.63333333 0.6375 0.64166667 0.64583333 0.65 0.65416667 0.65833333 0.6625 0.66666667 0.67083333 0.675 0.67916667 0.68333333 0.6875 0.69166667 0.69583333 0.7 0.70416667 0.70833333 0.7125 0.71666667 0.72083333 0.725 0.72916667 0.73333333 0.7375 0.74166667 0.74583333 0.75 0.75416667 0.75833333 0.7625 0.76666667 0.77083333 0.775 0.77916667 0.78333333 0.7875 0.79166667 0.79583333 0.8 0.80416667 0.80833333 0.8125 0.81666667 0.82083333 0.825 0.82916667 0.83333333 0.8375 0.84166667 0.84583333 0.85 0.85416667 0.85833333 0.8625 0.86666667 0.87083333 0.875 0.87916667 0.88333333 0.8875 0.89166667 0.89583333 0.9 0.90416667 0.90833333 0.9125 0.91666667 0.92083333 0.925 0.92916667 0.93333333 0.9375 0.94166667 0.94583333 0.95 0.95416667 0.95833333 0.9625 0.96666667 0.97083333 0.975 0.97916667 0.98333333 0.9875 0.99166667 0.99583333 1 1 1 1 1 1
  arc A5 (-0.3607, -6.6569) -> (0.3607, -6.6569) centre (0, 0) ccw
  spline S5 degree 5 poles (0.3607, -6.6569) (0.3623, -6.6549) (0.3655, -6.6508) (0.3702, -6.6447) (0.3766, -6.6365) (0.3845, -6.6263) (0.3923, -6.6161) (0.4001, -6.6059) (0.4079, -6.5957) (0.4156, -6.5855) (0.4232, -6.5754) (0.4308, -6.5652) (0.4384, -6.555) (0.4459, -6.5448) (0.4533, -6.5346) (0.4607, -6.5244) (0.4681, -6.5143) (0.4754, -6.5041) (0.4826, -6.4939) (0.4898, -6.4838) (0.497, -6.4736) (0.5041, -6.4634) (0.5112, -6.4533) (0.5182, -6.4431) (0.5252, -6.433) (0.5321, -6.4229) (0.5389, -6.4127) (0.5458, -6.4026) (0.5525, -6.3925) (0.5593, -6.3824) (0.5659, -6.3722) (0.5726, -6.3621) (0.5791, -6.3521) (0.5857, -6.342) (0.5921, -6.3319) (0.5986, -6.3218) (0.605, -6.3117) (0.6113, -6.3017) (0.6176, -6.2916) (0.6238, -6.2816) (0.63, -6.2716) (0.6362, -6.2616) (0.6423, -6.2515) (0.6483, -6.2415) (0.6543, -6.2316) (0.6602, -6.2216) (0.6661, -6.2116) (0.672, -6.2016) (0.6778, -6.1917) (0.6836, -6.1818) (0.6893, -6.1718) (0.6949, -6.1619) (0.7005, -6.152) (0.7061, -6.1421) (0.7116, -6.1323) (0.7171, -6.1224) (0.7225, -6.1126) (0.7279, -6.1027) (0.7332, -6.0929) (0.7385, -6.0831) (0.7437, -6.0733) (0.7489, -6.0635) (0.754, -6.0538) (0.7591, -6.044) (0.7642, -6.0343) (0.7692, -6.0246) (0.7741, -6.0149) (0.779, -6.0052) (0.7839, -5.9956) (0.7887, -5.9859) (0.7934, -5.9763) (0.7981, -5.9667) (0.8028, -5.9571) (0.8074, -5.9475) (0.812, -5.938) (0.8165, -5.9284) (0.821, -5.9189) (0.8254, -5.9094) (0.8298, -5.8999) (0.8341, -5.8905) (0.8384, -5.881) (0.8427, -5.8716) (0.8469, -5.8622) (0.851, -5.8529) (0.8551, -5.8435) (0.8592, -5.8342) (0.8632, -5.8249) (0.8672, -5.8156) (0.8711, -5.8063) (0.875, -5.7971) (0.8788, -5.7879) (0.8826, -5.7787) (0.8863, -5.7695) (0.89, -5.7604) (0.8937, -5.7513) (0.8973, -5.7422) (0.9008, -5.7331) (0.9044, -5.7241) (0.9078, -5.7151) (0.9113, -5.7061) (0.9146, -5.6971) (0.918, -5.6882) (0.9213, -5.6793) (0.9245, -5.6704) (0.9277, -5.6616) (0.9309, -5.6528) (0.934, -5.644) (0.9371, -5.6352) (0.9401, -5.6265) (0.9431, -5.6178) (0.946, -5.6091) (0.9489, -5.6005) (0.9518, -5.5919) (0.9546, -5.5833) (0.9574, -5.5747) (0.9601, -5.5662) (0.9628, -5.5577) (0.9654, -5.5493) (0.968, -5.5409) (0.9706, -5.5325) (0.9731, -5.5242) (0.9756, -5.5159) (0.978, -5.5076) (0.9804, -5.4993) (0.9828, -5.4911) (0.9851, -5.483) (0.9874, -5.4748) (0.9896, -5.4667) (0.9918, -5.4587) (0.9939, -5.4506) (0.996, -5.4427) (0.9981, -5.4347) (1.0001, -5.4268) (1.0021, -5.4189) (1.0041, -5.4111) (1.006, -5.4033) (1.0079, -5.3956) (1.0097, -5.3879) (1.0115, -5.3802) (1.0133, -5.3726) (1.015, -5.365) (1.0167, -5.3574) (1.0183, -5.3499) (1.0199, -5.3425) (1.0215, -5.3351) (1.023, -5.3277) (1.0245, -5.3204) (1.026, -5.3131) (1.0274, -5.3059) (1.0288, -5.2987) (1.0301, -5.2915) (1.0314, -5.2844) (1.0327, -5.2774) (1.034, -5.2704) (1.0352, -5.2634) (1.0364, -5.2565) (1.0375, -5.2496) (1.0386, -5.2428) (1.0397, -5.2361) (1.0407, -5.2294) (1.0417, -5.2227) (1.0427, -5.2161) (1.0436, -5.2095) (1.0446, -5.203) (1.0454, -5.1966) (1.0463, -5.1902) (1.0471, -5.1838) (1.0479, -5.1775) (1.0486, -5.1713) (1.0493, -5.1651) (1.05, -5.159) (1.0507, -5.1529) (1.0513, -5.1469) (1.0519, -5.1409) (1.0525, -5.135) (1.0531, -5.1291) (1.0536, -5.1234) (1.0541, -5.1176) (1.0545, -5.112) (1.055, -5.1063) (1.0554, -5.1008) (1.0558, -5.0953) (1.0561, -5.0899) (1.0565, -5.0845) (1.0568, -5.0792) (1.0571, -5.074) (1.0573, -5.0688) (1.0576, -5.0637) (1.0578, -5.0586) (1.058, -5.0536) (1.0581, -5.0487) (1.0583, -5.0439) (1.0584, -5.0391) (1.0585, -5.0344) (1.0586, -5.0297) (1.0587, -5.0251) (1.0587, -5.0206) (1.0587, -5.0162) (1.0587, -5.0118) (1.0587, -5.0075) (1.0587, -5.0033) (1.0587, -4.9992) (1.0586, -4.9951) (1.0585, -4.9911) (1.0584, -4.9872) (1.0583, -4.9833) (1.0582, -4.9795) (1.0581, -4.9758) (1.058, -4.9722) (1.0578, -4.9687) (1.0576, -4.9652) (1.0575, -4.9618) (1.0573, -4.9585) (1.0571, -4.9553) (1.0569, -4.9521) (1.0567, -4.9491) (1.0564, -4.9461) (1.0562, -4.9432) (1.056, -4.9404) (1.0558, -4.9377) (1.0555, -4.9351) (1.0553, -4.9325) (1.055, -4.9301) (1.0548, -4.9277) (1.0545, -4.9254) (1.0543, -4.9232) (1.054, -4.9211) (1.0538, -4.9191) (1.0536, -4.9172) (1.0533, -4.9154) (1.0531, -4.9137) (1.0529, -4.9121) (1.0526, -4.9106) (1.0524, -4.9092) (1.0522, -4.9078) (1.052, -4.9066) (1.0518, -4.9055) (1.0517, -4.9045) (1.0515, -4.9036) (1.0514, -4.9028) (1.0512, -4.9021) (1.0512, -4.9016) (1.0511, -4.9013) (1.0511, -4.9011) (1.051, -4.9011) knots -1 -1 -1 -1 -1 -1 -0.99583333 -0.99166667 -0.9875 -0.98333333 -0.97916667 -0.975 -0.97083333 -0.96666667 -0.9625 -0.95833333 -0.95416667 -0.95 -0.94583333 -0.94166667 -0.9375 -0.93333333 -0.92916667 -0.925 -0.92083333 -0.91666667 -0.9125 -0.90833333 -0.90416667 -0.9 -0.89583333 -0.89166667 -0.8875 -0.88333333 -0.87916667 -0.875 -0.87083333 -0.86666667 -0.8625 -0.85833333 -0.85416667 -0.85 -0.84583333 -0.84166667 -0.8375 -0.83333333 -0.82916667 -0.825 -0.82083333 -0.81666667 -0.8125 -0.80833333 -0.80416667 -0.8 -0.79583333 -0.79166667 -0.7875 -0.78333333 -0.77916667 -0.775 -0.77083333 -0.76666667 -0.7625 -0.75833333 -0.75416667 -0.75 -0.74583333 -0.74166667 -0.7375 -0.73333333 -0.72916667 -0.725 -0.72083333 -0.71666667 -0.7125 -0.70833333 -0.70416667 -0.7 -0.69583333 -0.69166667 -0.6875 -0.68333333 -0.67916667 -0.675 -0.67083333 -0.66666667 -0.6625 -0.65833333 -0.65416667 -0.65 -0.64583333 -0.64166667 -0.6375 -0.63333333 -0.62916667 -0.625 -0.62083333 -0.61666667 -0.6125 -0.60833333 -0.60416667 -0.6 -0.59583333 -0.59166667 -0.5875 -0.58333333 -0.57916667 -0.575 -0.57083333 -0.56666667 -0.5625 -0.55833333 -0.55416667 -0.55 -0.54583333 -0.54166667 -0.5375 -0.53333333 -0.52916667 -0.525 -0.52083333 -0.51666667 -0.5125 -0.50833333 -0.50416667 -0.5 -0.49583333 -0.49166667 -0.4875 -0.48333333 -0.47916667 -0.475 -0.47083333 -0.46666667 -0.4625 -0.45833333 -0.45416667 -0.45 -0.44583333 -0.44166667 -0.4375 -0.43333333 -0.42916667 -0.425 -0.42083333 -0.41666667 -0.4125 -0.40833333 -0.40416667 -0.4 -0.39583333 -0.39166667 -0.3875 -0.38333333 -0.37916667 -0.375 -0.37083333 -0.36666667 -0.3625 -0.35833333 -0.35416667 -0.35 -0.34583333 -0.34166667 -0.3375 -0.33333333 -0.32916667 -0.325 -0.32083333 -0.31666667 -0.3125 -0.30833333 -0.30416667 -0.3 -0.29583333 -0.29166667 -0.2875 -0.28333333 -0.27916667 -0.275 -0.27083333 -0.26666667 -0.2625 -0.25833333 -0.25416667 -0.25 -0.24583333 -0.24166667 -0.2375 -0.23333333 -0.22916667 -0.225 -0.22083333 -0.21666667 -0.2125 -0.20833333 -0.20416667 -0.2 -0.19583333 -0.19166667 -0.1875 -0.18333333 -0.17916667 -0.175 -0.17083333 -0.16666667 -0.1625 -0.15833333 -0.15416667 -0.15 -0.14583333 -0.14166667 -0.1375 -0.13333333 -0.12916667 -0.125 -0.12083333 -0.11666667 -0.1125 -0.10833333 -0.10416667 -0.1 -0.09583333 -0.09166667 -0.0875 -0.08333333 -0.07916667 -0.075 -0.07083333 -0.06666667 -0.0625 -0.05833333 -0.05416667 -0.05 -0.04583333 -0.04166667 -0.0375 -0.03333333 -0.02916667 -0.025 -0.02083333 -0.01666667 -0.0125 -0.00833333 -0.00416667 0 0 0 0 0 0
  line L10 (1.051, -4.9011) -> (1.0509, -4.9003)
  line L11 (1.0509, -4.9003) -> (0.7688, -3.5852)
  arc A6 (0.7688, -3.5852) -> (1.9914, -3.0787) centre (0, 0) ccw
  line L12 (1.9914, -3.0787) -> (2.7219, -4.2081)
  line L13 (2.7219, -4.2081) -> (2.7224, -4.2088)
  spline S6 degree 5 poles (2.7224, -4.2088) (2.7224, -4.2088) (2.7225, -4.209) (2.7227, -4.2093) (2.723, -4.2096) (2.7234, -4.2102) (2.7238, -4.2109) (2.7244, -4.2116) (2.725, -4.2125) (2.7256, -4.2134) (2.7263, -4.2144) (2.7271, -4.2155) (2.728, -4.2166) (2.7289, -4.2179) (2.7299, -4.2192) (2.7309, -4.2205) (2.732, -4.222) (2.7332, -4.2235) (2.7345, -4.2251) (2.7358, -4.2267) (2.7371, -4.2285) (2.7386, -4.2302) (2.7401, -4.2321) (2.7416, -4.234) (2.7433, -4.236) (2.7449, -4.238) (2.7467, -4.2401) (2.7485, -4.2422) (2.7504, -4.2444) (2.7524, -4.2467) (2.7544, -4.249) (2.7564, -4.2514) (2.7586, -4.2538) (2.7608, -4.2563) (2.7631, -4.2588) (2.7654, -4.2613) (2.7678, -4.264) (2.7702, -4.2666) (2.7728, -4.2693) (2.7754, -4.2721) (2.778, -4.2749) (2.7807, -4.2777) (2.7835, -4.2806) (2.7863, -4.2835) (2.7893, -4.2865) (2.7922, -4.2895) (2.7953, -4.2925) (2.7984, -4.2956) (2.8015, -4.2987) (2.8047, -4.3019) (2.808, -4.3051) (2.8114, -4.3083) (2.8148, -4.3116) (2.8182, -4.3149) (2.8218, -4.3182) (2.8254, -4.3216) (2.829, -4.3249) (2.8328, -4.3284) (2.8365, -4.3318) (2.8404, -4.3353) (2.8443, -4.3388) (2.8483, -4.3423) (2.8523, -4.3459) (2.8564, -4.3495) (2.8605, -4.3531) (2.8648, -4.3567) (2.869, -4.3604) (2.8734, -4.364) (2.8778, -4.3678) (2.8822, -4.3715) (2.8867, -4.3752) (2.8913, -4.379) (2.896, -4.3828) (2.9007, -4.3866) (2.9054, -4.3904) (2.9103, -4.3943) (2.9152, -4.3981) (2.9201, -4.402) (2.9251, -4.4059) (2.9302, -4.4098) (2.9353, -4.4138) (2.9405, -4.4177) (2.9457, -4.4217) (2.951, -4.4256) (2.9564, -4.4296) (2.9618, -4.4336) (2.9673, -4.4376) (2.9728, -4.4416) (2.9784, -4.4457) (2.9841, -4.4497) (2.9898, -4.4538) (2.9956, -4.4578) (3.0014, -4.4619) (3.0073, -4.466) (3.0133, -4.4701) (3.0193, -4.4742) (3.0253, -4.4783) (3.0314, -4.4824) (3.0376, -4.4865) (3.0439, -4.4906) (3.0502, -4.4948) (3.0565, -4.4989) (3.0629, -4.503) (3.0694, -4.5072) (3.0759, -4.5113) (3.0825, -4.5155) (3.0891, -4.5196) (3.0958, -4.5238) (3.1026, -4.5279) (3.1094, -4.5321) (3.1162, -4.5362) (3.1231, -4.5404) (3.1301, -4.5445) (3.1371, -4.5487) (3.1442, -4.5529) (3.1514, -4.557) (3.1586, -4.5612) (3.1658, -4.5653) (3.1731, -4.5695) (3.1805, -4.5736) (3.1879, -4.5777) (3.1953, -4.5819) (3.2029, -4.586) (3.2104, -4.5902) (3.2181, -4.5943) (3.2258, -4.5984) (3.2335, -4.6025) (3.2413, -4.6066) (3.2491, -4.6107) (3.257, -4.6148) (3.265, -4.6189) (3.273, -4.623) (3.281, -4.6271) (3.2891, -4.6311) (3.2973, -4.6352) (3.3055, -4.6392) (3.3138, -4.6433) (3.3221, -4.6473) (3.3304, -4.6513) (3.3389, -4.6553) (3.3473, -4.6593) (3.3559, -4.6633) (3.3644, -4.6673) (3.3731, -4.6713) (3.3817, -4.6752) (3.3905, -4.6792) (3.3992, -4.6831) (3.4081, -4.687) (3.4169, -4.6909) (3.4259, -4.6948) (3.4348, -4.6987) (3.4439, -4.7026) (3.4529, -4.7064) (3.4621, -4.7102) (3.4712, -4.7141) (3.4805, -4.7179) (3.4897, -4.7217) (3.4991, -4.7254) (3.5084, -4.7292) (3.5178, -4.7329) (3.5273, -4.7367) (3.5368, -4.7404) (3.5464, -4.7441) (3.556, -4.7477) (3.5657, -4.7514) (3.5754, -4.755) (3.5851, -4.7586) (3.5949, -4.7622) (3.6048, -4.7658) (3.6147, -4.7694) (3.6246, -4.7729) (3.6346, -4.7765) (3.6446, -4.78) (3.6547, -4.7834) (3.6648, -4.7869) (3.675, -4.7904) (3.6852, -4.7938) (3.6955, -4.7972) (3.7058, -4.8006) (3.7161, -4.8039) (3.7265, -4.8073) (3.737, -4.8106) (3.7475, -4.8139) (3.758, -4.8171) (3.7686, -4.8204) (3.7792, -4.8236) (3.7899, -4.8268) (3.8006, -4.83) (3.8113, -4.8331) (3.8221, -4.8363) (3.833, -4.8394) (3.8439, -4.8424) (3.8548, -4.8455) (3.8658, -4.8485) (3.8768, -4.8515) (3.8878, -4.8545) (3.8989, -4.8575) (3.9101, -4.8604) (3.9212, -4.8633) (3.9325, -4.8662) (3.9437, -4.869) (3.955, -4.8719) (3.9664, -4.8747) (3.9778, -4.8774) (3.9892, -4.8802) (4.0007, -4.8829) (4.0122, -4.8856) (4.0237, -4.8882) (4.0353, -4.8909) (4.0469, -4.8935) (4.0586, -4.896) (4.0703, -4.8986) (4.0821, -4.9011) (4.0939, -4.9036) (4.1057, -4.906) (4.1176, -4.9085) (4.1295, -4.9109) (4.1414, -4.9132) (4.1534, -4.9156) (4.1654, -4.9179) (4.1775, -4.9201) (4.1896, -4.9224) (4.2017, -4.9246) (4.2139, -4.9268) (4.2261, -4.9289) (4.2383, -4.9311) (4.2506, -4.9332) (4.2629, -4.9352) (4.2753, -4.9372) (4.2877, -4.9392) (4.3001, -4.9412) (4.3126, -4.9431) (4.3251, -4.945) (4.3377, -4.9469) (4.3502, -4.9487) (4.3628, -4.9505) (4.3755, -4.9523) (4.3882, -4.954) (4.4009, -4.9557) (4.4136, -4.9574) (4.4264, -4.959) (4.4367, -4.9603) (4.4444, -4.9612) (4.4495, -4.9619) (4.4521, -4.9622) knots 0 0 0 0 0 0 0.00416667 0.00833333 0.0125 0.01666667 0.02083333 0.025 0.02916667 0.03333333 0.0375 0.04166667 0.04583333 0.05 0.05416667 0.05833333 0.0625 0.06666667 0.07083333 0.075 0.07916667 0.08333333 0.0875 0.09166667 0.09583333 0.1 0.10416667 0.10833333 0.1125 0.11666667 0.12083333 0.125 0.12916667 0.13333333 0.1375 0.14166667 0.14583333 0.15 0.15416667 0.15833333 0.1625 0.16666667 0.17083333 0.175 0.17916667 0.18333333 0.1875 0.19166667 0.19583333 0.2 0.20416667 0.20833333 0.2125 0.21666667 0.22083333 0.225 0.22916667 0.23333333 0.2375 0.24166667 0.24583333 0.25 0.25416667 0.25833333 0.2625 0.26666667 0.27083333 0.275 0.27916667 0.28333333 0.2875 0.29166667 0.29583333 0.3 0.30416667 0.30833333 0.3125 0.31666667 0.32083333 0.325 0.32916667 0.33333333 0.3375 0.34166667 0.34583333 0.35 0.35416667 0.35833333 0.3625 0.36666667 0.37083333 0.375 0.37916667 0.38333333 0.3875 0.39166667 0.39583333 0.4 0.40416667 0.40833333 0.4125 0.41666667 0.42083333 0.425 0.42916667 0.43333333 0.4375 0.44166667 0.44583333 0.45 0.45416667 0.45833333 0.4625 0.46666667 0.47083333 0.475 0.47916667 0.48333333 0.4875 0.49166667 0.49583333 0.5 0.50416667 0.50833333 0.5125 0.51666667 0.52083333 0.525 0.52916667 0.53333333 0.5375 0.54166667 0.54583333 0.55 0.55416667 0.55833333 0.5625 0.56666667 0.57083333 0.575 0.57916667 0.58333333 0.5875 0.59166667 0.59583333 0.6 0.60416667 0.60833333 0.6125 0.61666667 0.62083333 0.625 0.62916667 0.63333333 0.6375 0.64166667 0.64583333 0.65 0.65416667 0.65833333 0.6625 0.66666667 0.67083333 0.675 0.67916667 0.68333333 0.6875 0.69166667 0.69583333 0.7 0.70416667 0.70833333 0.7125 0.71666667 0.72083333 0.725 0.72916667 0.73333333 0.7375 0.74166667 0.74583333 0.75 0.75416667 0.75833333 0.7625 0.76666667 0.77083333 0.775 0.77916667 0.78333333 0.7875 0.79166667 0.79583333 0.8 0.80416667 0.80833333 0.8125 0.81666667 0.82083333 0.825 0.82916667 0.83333333 0.8375 0.84166667 0.84583333 0.85 0.85416667 0.85833333 0.8625 0.86666667 0.87083333 0.875 0.87916667 0.88333333 0.8875 0.89166667 0.89583333 0.9 0.90416667 0.90833333 0.9125 0.91666667 0.92083333 0.925 0.92916667 0.93333333 0.9375 0.94166667 0.94583333 0.95 0.95416667 0.95833333 0.9625 0.96666667 0.97083333 0.975 0.97916667 0.98333333 0.9875 0.99166667 0.99583333 1 1 1 1 1 1
  arc A7 (4.4521, -4.9622) -> (4.9622, -4.4521) centre (0, 0) ccw